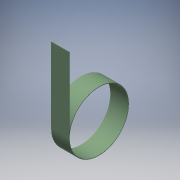
# Autodesk Inventor part: FoilCoil2
Saved by Autodesk Inventor 2019 (Build 230136000, 136)
## iProperties
Created: 2017-01-18
Part Number: FoilCoil2
Document SubType Name: Modeling
Designer: Administrator
Density: 1 g/cm^3
Mass: 0.103056 g
Surface Area: 10.5803 cm^2
Volume: 0.103056 cm^3
Material: Generic
Appearance: Green Pastel
Author: Administrator
Autodesk Inventor part; units mm, degrees
ref_plane "YZ Plane" through (0, 0, 0) normal (1, 0, 0) x (0, 1, 0)
ref_plane "XZ Plane" through (0, 0, 0) normal (0, 1, 0) x (-1, 0, 0)
ref_plane "XY Plane" through (0, 0, 0) normal (0, 0, 1) x (1, 0, 0)
sketch "Sketch1" plane through (0, 0, 0) normal (0, 0, 1) x (1, 0, 0)
  line L0 (0, 0) -> (6, 0)
  line L1 (6, 0) -> (6, 0.2)
  line L2 (6, 0.2) -> (0, 0.2)
  line L3 (0, 0.2) -> (0, 0)
  dimension "d0" = 0.2
  dimension "d1" = 6
  constraints: 8 end point, 2 parallel, 1 horizontal, 1 perpendicular, 1 other
  measures "d0" distance of L0.end L1.end
  measures "d1" distance of L0.start L0.end
extrude "Extrusion1" add sketch "Sketch1" along normal blind 10
sketch "Sketch2" plane through (0, 0, 0) normal (1, 0, 0) x (0, 1, 0)
  line L0 (0, 0) -> (0.2, 0) projected
  line L1 (0, 0) -> (10, 0)
  circle A0 centre (10, 0) radius 10
  circle A1 centre (10, 0) radius 9.8
  dimension "d4" = 10
  constraints: 2 coincident, 2 end point, 2 horizontal alignment, 1 collinear, 4 other
  measures "d4" distance of L0.start L1.end
extrude "Extrusion2" add sketch "Sketch2" along normal up to surface (6 mm away)
sketch "Sketch3" plane through (0, 0, 10) normal (0, 0, 1) x (1, 0, 0)
  line L0 (0, 0) -> (0, 0.2) projected
  line L1 (6, 0) -> (0, 0) projected
  line L2 (6, 0.2) -> (6, 0) projected
  line L3 (0, 0.2) -> (6, 0.2) projected
extrude "Extrusion3" add sketch "Sketch3" along normal blind 15
body "Solid1"
